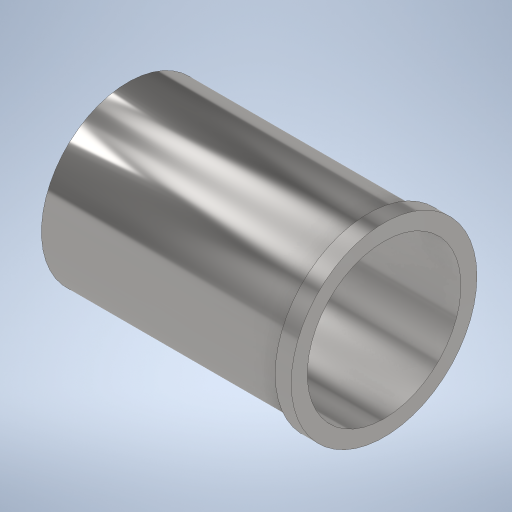
# Autodesk Inventor part: fitting
Saved by Autodesk Inventor 2024 (Build 280153000, 153)
## iProperties
Created: 2024-03-08
Part Number: fitting
Material: Stahl, hochfest, niedrig legiert
Document SubType Name: Modeling
Designer: ffogue
Density: 7.85 g/cm^3
Appearance: Stahl - poliert
Author: ffogue
Autodesk Inventor part; units mm, degrees
ref_plane "YZ Plane" through (0, 0, 0) normal (1, 0, 0) x (0, 1, 0)
ref_plane "XZ Plane" through (0, 0, 0) normal (0, 1, 0) x (-1, 0, 0)
ref_plane "XY Plane" through (0, 0, 0) normal (0, 0, 1) x (1, 0, 0)
sketch "Skizze1" plane through (0, 0, 0) normal (0, 0, 1) x (1, 0, 0)
  line L0 (0, 0) -> (40, 0)
  line L1 (0, 0) -> (0, 13.5)
  line L2 (0, 13.5) -> (37.5, 13.5)
  line L3 (37.5, 13.5) -> (37.5, 14.5)
  line L4 (37.5, 14.5) -> (40, 14.5)
  line L5 (40, 14.5) -> (40, 0)
  dimension "d0" = 29
  dimension "d1" = 27
  dimension "d2" = 2.5
  dimension "d3" = 37.5
  constraints: 12 end point, 4 perpendicular, 1 horizontal, 1 vertical
  measures "d0" diameter of L4 L0
  measures "d1" diameter of L2 L0
  measures "d2" distance between parallel lines of L5 L3
  measures "d3" distance between parallel lines of L3 L1
revolve "Umdrehung1" add sketch "Skizze1" angle 360 about axis through (0, 0, 0) along (1, 0, 0)
sketch "Skizze2" plane through (0, 0, 0) normal (-1, 0, 0) x (0, 0, 1)
  circle A0 centre (0, 0) radius 13.5 projected
  constraints: 1 coincident
hole "Bohrung1" at (0, 0, 0) direction (1, 0, 0) diameter 24 end through all
